Autodesk Inventor part; units mm, degrees
(part 2 of 2)
  arc A620 (20.4911, 0.6052) -> (20.4754, 1.0044) centre (0, 0) ccw
  arc A621 (20.3804, 2.2111) -> (20.3335, 2.6078) centre (0, 0) ccw
  arc A622 (20.1441, 3.8033) -> (20.0662, 4.1951) centre (0, 0) ccw
  arc A623 (19.7836, 5.372) -> (19.6752, 5.7565) centre (0, 0) ccw
  arc A624 (19.3011, 6.9077) -> (19.1629, 7.2825) centre (0, 0) ccw
  arc A625 (18.6997, 8.4007) -> (18.5324, 8.7635) centre (0, 0) ccw
  arc A626 (17.9829, 9.842) -> (17.7877, 10.1905) centre (0, 0) ccw
  arc A627 (17.1553, 11.2226) -> (16.9334, 11.5547) centre (0, 0) ccw
  arc A628 (16.2219, 12.534) -> (15.9746, 12.8477) centre (0, 0) ccw
  arc A629 (15.1885, 13.7681) -> (14.9173, 14.0614) centre (0, 0) ccw
  arc A630 (14.0614, 14.9173) -> (13.7681, 15.1885) centre (0, 0) ccw
  arc A631 (12.8477, 15.9746) -> (12.534, 16.2219) centre (0, 0) ccw
  arc A632 (11.5547, 16.9334) -> (11.2226, 17.1553) centre (0, 0) ccw
  arc A633 (10.1905, 17.7877) -> (9.842, 17.9829) centre (0, 0) ccw
  arc A634 (8.7635, 18.5324) -> (8.4007, 18.6997) centre (0, 0) ccw
  arc A635 (7.2825, 19.1629) -> (6.9077, 19.3011) centre (0, 0) ccw
  arc A636 (5.7565, 19.6752) -> (5.372, 19.7836) centre (0, 0) ccw
  arc A637 (4.1951, 20.0662) -> (3.8033, 20.1441) centre (0, 0) ccw
  arc A638 (2.6078, 20.3335) -> (2.2111, 20.3804) centre (0, 0) ccw
  arc A639 (1.0044, 20.4754) -> (0.6052, 20.4911) centre (0, 0) ccw
  line L0 (-22.5, 0) -> (22.5, 0)
  line L1 (0, -22.5) -> (0, 22.5)
  point P0 (0, 0)
  constraints: 960 point on circle, 480 centre point, 4 end point, 2 horizontal alignment, 2 vertical alignment, 1 horizontal, 1 vertical, 2081 other
extrude "押し出し1" add sketch "スケッチ1" along normal blind 3
sketch "スケッチ6" plane through (0, 0, 0) normal (0, 1, 0) x (-1, 0, 0)
  line L0 (0, 0) -> (0, 3)
  line L1 (0, 3) -> (-20, 3)
  line L2 (0, 0) -> (-20, 0)
  line L3 (-20, 3) -> (-20.5, 2.5)
  line L4 (-20.5, 2.5) -> (-20.5, 0.5)
  line L5 (-20.5, 0.5) -> (-20, 0)
  line L6 (-20, 3) -> (-20.5, 3)
  line L7 (-20.5, 3) -> (-20.5, 2.5)
  line L8 (-20, 0) -> (-20.5, 0)
  line L9 (-20.5, 0) -> (-20.5, 0.5)
  line L10 (0, 3) -> (0, 0)
  dimension "d30" = 3
  dimension "d31" = 0.5
  dimension "d32" = 0.5
  dimension "d33" = 0.5
  dimension "d34" = 0.5
  dimension "d35" = 20.5
  constraints: 22 end point, 4 horizontal, 3 vertical, 1 vertical alignment
  measures "d30" distance of L0.start L0.end
  measures "d31" horizontal distance of L1.end L3.end
  measures "d32" horizontal distance of L1.end L3.end
  measures "d33" horizontal distance of L4.end L2.end
  measures "d34" horizontal distance of L4.end L2.end
  measures "d35" distance from line of L0.start L4
revolve "回転1" cut sketch "スケッチ6" angle 360 about axis through (0, 0, 0) along (0, 0, 1) contours L8 L9 L5 | L3 L7 L6
sketch "スケッチ7" plane through (0, 0, 3) normal (0, 0, 1) x (1, 0, 0)
  circle A0 centre (0, 0) radius 17.25
  dimension "d37" = 34.5
  constraints: 1 centre point, 1 coincident
  measures "d37" diameter of A0
extrude "押し出し6" cut sketch "スケッチ7" against normal blind 0.8
sketch "スケッチ8" plane through (0, 0, 0) normal (0, 0, -1) x (-1, 0, 0)
  arc A0 (-0.3926, 19.9961) -> (-1.1774, 19.9653) centre (0, 0) ccw projected
  arc A1 (-1.1774, 19.9653) -> (-1.2665, 19.6357) centre (4.9618, 18.1301) ccw projected
  arc A2 (-1.2665, 19.6357) -> (-1.331, 19.3292) centre (3.8577, 18.3965) ccw projected
  arc A3 (-1.331, 19.3292) -> (-1.7091, 19.2995) centre (0, 0) ccw projected
  arc A4 (-1.7091, 19.2995) -> (-1.8197, 19.5895) centre (-6.6881, 17.5665) ccw projected
  arc A5 (-1.8197, 19.5895) -> (-1.9603, 19.9037) centre (-7.7369, 17.1307) ccw projected
  arc A6 (-1.9603, 19.9037) -> (-2.7403, 19.8114) centre (0, 0) ccw projected
  arc A7 (-2.7403, 19.8114) -> (-2.8032, 19.4758) centre (3.5241, 18.4635) ccw projected
  arc A8 (-2.8032, 19.4758) -> (-2.8435, 19.1652) centre (2.4025, 18.6425) ccw projected
  arc A9 (-2.8435, 19.1652) -> (-3.2181, 19.1059) centre (0, 0) ccw projected
  arc A10 (-3.2181, 19.1059) -> (-3.3511, 19.3863) centre (-8.0457, 16.9876) ccw projected
  arc A11 (-3.3511, 19.3863) -> (-3.5159, 19.6885) centre (-9.0571, 16.4708) ccw projected
  arc A12 (-3.5159, 19.6885) -> (-4.2862, 19.5353) centre (0, 0) ccw projected
  arc A13 (-4.2862, 19.5353) -> (-4.3226, 19.1958) centre (2.0646, 18.6831) ccw projected
  arc A14 (-4.3226, 19.1958) -> (-4.3384, 18.883) centre (0.9324, 18.7735) ccw projected
  arc A15 (-4.3384, 18.883) -> (-4.7072, 18.7945) centre (0, 0) ccw projected
  arc A16 (-4.7072, 18.7945) -> (-4.8632, 19.066) centre (-9.3537, 16.304) ccw projected
  arc A17 (-4.8632, 19.066) -> (-5.0498, 19.352) centre (-10.3215, 15.7095) ccw projected
  arc A18 (-5.0498, 19.352) -> (-5.8057, 19.1388) centre (0, 0) ccw projected
  arc A19 (-5.8057, 19.1388) -> (-5.8154, 18.7975) centre (0.5924, 18.7875) ccw projected
  arc A20 (-5.8154, 18.7975) -> (-5.8066, 18.4844) centre (-0.5434, 18.7888) ccw projected
  arc A21 (-5.8066, 18.4844) -> (-6.1673, 18.3672) centre (0, 0) ccw projected
  arc A22 (-6.1673, 18.3672) -> (-6.3442, 18.6257) centre (-10.6041, 15.5199) ccw projected
  arc A23 (-6.3442, 18.6257) -> (-6.5526, 18.8961) centre (-11.5222, 14.8512) ccw projected
  arc A24 (-6.5526, 18.8961) -> (-7.2894, 18.6243) centre (0, 0) ccw projected
  arc A25 (-7.2894, 18.6243) -> (-7.2723, 18.2833) centre (-0.8835, 18.776) ccw projected
  arc A26 (-7.2723, 18.2833) -> (-7.2389, 17.9719) centre (-2.0159, 18.6882) ccw projected
  arc A27 (-7.2389, 17.9719) -> (-7.5893, 17.8267) centre (0, 0) ccw projected
  arc A28 (-7.5893, 17.8267) -> (-7.786, 18.0705) centre (-11.7891, 14.64) ccw projected
  arc A29 (-7.786, 18.0705) -> (-8.0149, 18.3238) centre (-12.6519, 13.9014) ccw projected
  arc A30 (-8.0149, 18.3238) -> (-8.7282, 17.995) centre (0, 0) ccw projected
  arc A31 (-8.7282, 17.995) -> (-8.6843, 17.6563) centre (-2.3539, 18.6488) ccw projected
  arc A32 (-8.6843, 17.6563) -> (-8.6267, 17.3485) centre (-3.476, 18.4724) ccw projected
  arc A33 (-8.6267, 17.3485) -> (-8.9646, 17.1763) centre (0, 0) ccw projected
  arc A34 (-8.9646, 17.1763) -> (-9.1797, 17.4039) centre (-12.9014, 13.6699) ccw projected
  arc A35 (-9.1797, 17.4039) -> (-9.4279, 17.6384) centre (-13.7036, 12.8659) ccw projected
  arc A36 (-9.4279, 17.6384) -> (-10.1132, 17.2547) centre (0, 0) ccw projected
  arc A37 (-10.1132, 17.2547) -> (-10.0429, 16.9205) centre (-3.8099, 18.4067) ccw projected
  arc A38 (-10.0429, 16.9205) -> (-9.9612, 16.6182) centre (-4.9146, 18.1428) ccw projected
  arc A39 (-9.9612, 16.6182) -> (-10.2846, 16.42) centre (0, 0) ccw projected
  arc A40 (-10.2846, 16.42) -> (-10.5169, 16.63) centre (-13.9341, 12.6156) ccw projected
  arc A41 (-10.5169, 16.63) -> (-10.7827, 16.8444) centre (-14.6708, 11.7511) ccw projected
  arc A42 (-10.7827, 16.8444) -> (-11.4358, 16.408) centre (0, 0) ccw projected
  arc A43 (-11.4358, 16.408) -> (-11.3395, 16.0804) centre (-5.2423, 18.051) ccw projected
  arc A44 (-11.3395, 16.0804) -> (-11.2344, 15.7854) centre (-6.3229, 17.7012) ccw projected
  arc A45 (-11.2344, 15.7854) -> (-11.5412, 15.5625) centre (0, 0) ccw projected
  arc A46 (-11.5412, 15.5625) -> (-11.7893, 15.7536) centre (-14.881, 11.4834) ccw projected
  arc A47 (-11.7893, 15.7536) -> (-12.0711, 15.9464) centre (-15.5476, 10.5638) ccw projected
  arc A48 (-12.0711, 15.9464) -> (-12.6879, 15.4602) centre (0, 0) ccw projected
  arc A49 (-12.6879, 15.4602) -> (-12.5662, 15.1412) centre (-6.6424, 17.5841) ccw projected
  arc A50 (-12.5662, 15.1412) -> (-12.4383, 14.8553) centre (-7.6922, 17.1506) ccw projected
  arc A51 (-12.4383, 14.8553) -> (-12.7266, 14.609) centre (0, 0) ccw projected
  arc A52 (-12.7266, 14.609) -> (-12.989, 14.7801) centre (-15.7361, 10.2805) ccw projected
  arc A53 (-12.989, 14.7801) -> (-13.285, 14.9502) centre (-16.3285, 9.3114) ccw projected
  arc A54 (-13.285, 14.9502) -> (-13.8618, 14.417) centre (0, 0) ccw projected
  arc A55 (-13.8618, 14.417) -> (-13.7154, 14.1086) centre (-8.0015, 17.0087) ccw projected
  arc A56 (-13.7154, 14.1086) -> (-13.5655, 13.8336) centre (-9.0141, 16.4942) ccw projected
  arc A57 (-13.5655, 13.8336) -> (-13.8336, 13.5655) centre (0, 0) ccw projected
  arc A58 (-13.8336, 13.5655) -> (-14.1086, 13.7154) centre (-16.4942, 9.0141) ccw projected
  arc A59 (-14.1086, 13.7154) -> (-14.417, 13.8618) centre (-17.0087, 8.0015) ccw projected
  arc A60 (-14.417, 13.8618) -> (-14.9502, 13.285) centre (0, 0) ccw projected
  arc A61 (-14.9502, 13.285) -> (-14.7801, 12.989) centre (-9.3114, 16.3285) ccw projected
  arc A62 (-14.7801, 12.989) -> (-14.609, 12.7266) centre (-10.2805, 15.7361) ccw projected
  arc A63 (-14.609, 12.7266) -> (-14.8553, 12.4383) centre (0, 0) ccw projected
  arc A64 (-14.8553, 12.4383) -> (-15.1412, 12.5662) centre (-17.1506, 7.6922) ccw projected
  arc A65 (-15.1412, 12.5662) -> (-15.4602, 12.6879) centre (-17.5841, 6.6424) ccw projected
  arc A66 (-15.4602, 12.6879) -> (-15.9464, 12.0711) centre (0, 0) ccw projected
  arc A67 (-15.9464, 12.0711) -> (-15.7536, 11.7893) centre (-10.5638, 15.5476) ccw projected
  arc A68 (-15.7536, 11.7893) -> (-15.5625, 11.5412) centre (-11.4834, 14.881) ccw projected
  arc A69 (-15.5625, 11.5412) -> (-15.7854, 11.2344) centre (0, 0) ccw projected
  arc A70 (-15.7854, 11.2344) -> (-16.0804, 11.3395) centre (-17.7012, 6.3229) ccw projected
  arc A71 (-16.0804, 11.3395) -> (-16.408, 11.4358) centre (-18.051, 5.2423) ccw projected
  arc A72 (-16.408, 11.4358) -> (-16.8444, 10.7827) centre (0, 0) ccw projected
  arc A73 (-16.8444, 10.7827) -> (-16.63, 10.5169) centre (-11.7511, 14.6708) ccw projected
  arc A74 (-16.63, 10.5169) -> (-16.42, 10.2846) centre (-12.6156, 13.9341) ccw projected
  arc A75 (-16.42, 10.2846) -> (-16.6182, 9.9612) centre (0, 0) ccw projected
  arc A76 (-16.6182, 9.9612) -> (-16.9205, 10.0429) centre (-18.1428, 4.9146) ccw projected
  arc A77 (-16.9205, 10.0429) -> (-17.2547, 10.1132) centre (-18.4067, 3.8099) ccw projected
  arc A78 (-17.2547, 10.1132) -> (-17.6384, 9.4279) centre (0, 0) ccw projected
  arc A79 (-17.6384, 9.4279) -> (-17.4039, 9.1797) centre (-12.8659, 13.7036) ccw projected
  arc A80 (-17.4039, 9.1797) -> (-17.1763, 8.9646) centre (-13.6699, 12.9014) ccw projected
  arc A81 (-17.1763, 8.9646) -> (-17.3485, 8.6267) centre (0, 0) ccw projected
  arc A82 (-17.3485, 8.6267) -> (-17.6563, 8.6843) centre (-18.4724, 3.476) ccw projected
  arc A83 (-17.6563, 8.6843) -> (-17.995, 8.7282) centre (-18.6488, 2.3539) ccw projected
  arc A84 (-17.995, 8.7282) -> (-18.3238, 8.0149) centre (0, 0) ccw projected
  arc A85 (-18.3238, 8.0149) -> (-18.0705, 7.786) centre (-13.9014, 12.6519) ccw projected
  arc A86 (-18.0705, 7.786) -> (-17.8267, 7.5893) centre (-14.64, 11.7891) ccw projected
  arc A87 (-17.8267, 7.5893) -> (-17.9719, 7.2389) centre (0, 0) ccw projected
  arc A88 (-17.9719, 7.2389) -> (-18.2833, 7.2723) centre (-18.6882, 2.0159) ccw projected
  arc A89 (-18.2833, 7.2723) -> (-18.6243, 7.2894) centre (-18.776, 0.8835) ccw projected
  arc A90 (-18.6243, 7.2894) -> (-18.8961, 6.5526) centre (0, 0) ccw projected
  arc A91 (-18.8961, 6.5526) -> (-18.6234, 6.3425) centre (-14.8512, 11.5222) ccw projected
  arc A92 (-18.6234, 6.3425) -> (-18.3672, 6.1673) centre (-15.5198, 10.6041) ccw projected
  arc A93 (-18.3672, 6.1673) -> (-18.4844, 5.8066) centre (0, 0) ccw projected
  arc A94 (-18.4844, 5.8066) -> (-18.7975, 5.8154) centre (-18.7888, 0.5434) ccw projected
  arc A95 (-18.7975, 5.8154) -> (-19.1388, 5.8057) centre (-18.7875, -0.5924) ccw projected
  arc A96 (-19.1388, 5.8057) -> (-19.352, 5.0498) centre (0, 0) ccw projected
  arc A97 (-19.352, 5.0498) -> (-19.066, 4.8632) centre (-15.7095, 10.3215) ccw projected
  arc A98 (-19.066, 4.8632) -> (-18.7945, 4.7072) centre (-16.304, 9.3537) ccw projected
  arc A99 (-18.7945, 4.7072) -> (-18.883, 4.3384) centre (0, 0) ccw projected
  arc A100 (-18.883, 4.3384) -> (-19.1958, 4.3226) centre (-18.7735, -0.9324) ccw projected
  arc A101 (-19.1958, 4.3226) -> (-19.5353, 4.2862) centre (-18.6831, -2.0646) ccw projected
  arc A102 (-19.5353, 4.2862) -> (-19.6885, 3.5159) centre (0, 0) ccw projected
  arc A103 (-19.6885, 3.5159) -> (-19.3863, 3.3511) centre (-16.4708, 9.0571) ccw projected
  arc A104 (-19.3863, 3.3511) -> (-19.1059, 3.2181) centre (-16.9876, 8.0457) ccw projected
  arc A105 (-19.1059, 3.2181) -> (-19.1652, 2.8435) centre (0, 0) ccw projected
  arc A106 (-19.1652, 2.8435) -> (-19.4758, 2.8032) centre (-18.6425, -2.4025) ccw projected
  arc A107 (-19.4758, 2.8032) -> (-19.8114, 2.7403) centre (-18.4635, -3.5241) ccw projected
  arc A108 (-19.8114, 2.7403) -> (-19.9037, 1.9603) centre (0, 0) ccw projected
  arc A109 (-19.9037, 1.9603) -> (-19.592, 1.8208) centre (-17.1307, 7.7369) ccw projected
  arc A110 (-19.592, 1.8208) -> (-19.2995, 1.7091) centre (-17.5665, 6.6881) ccw projected
  arc A111 (-19.2995, 1.7091) -> (-19.3292, 1.331) centre (0, 0) ccw projected
  arc A112 (-19.3292, 1.331) -> (-19.6357, 1.2665) centre (-18.3965, -3.8577) ccw projected
  arc A113 (-19.6357, 1.2665) -> (-19.9653, 1.1774) centre (-18.1301, -4.9618) ccw projected
  arc A114 (-19.9653, 1.1774) -> (-19.9961, 0.3926) centre (0, 0) ccw projected
  arc A115 (-19.9961, 0.3926) -> (-19.6745, 0.278) centre (-17.6849, 6.369) ccw projected
  arc A116 (-19.6745, 0.278) -> (-19.3741, 0.1896) centre (-18.0371, 5.2892) ccw projected
  arc A117 (-19.3741, 0.1896) -> (-19.3741, -0.1896) centre (0, 0) ccw projected
  arc A118 (-19.3741, -0.1896) -> (-19.6745, -0.278) centre (-18.0371, -5.2892) ccw projected
  arc A119 (-19.6745, -0.278) -> (-19.9961, -0.3926) centre (-17.6849, -6.369) ccw projected
  arc A120 (-19.9961, -0.3926) -> (-19.9653, -1.1774) centre (0, 0) ccw projected
  arc A121 (-19.9653, -1.1774) -> (-19.6357, -1.2665) centre (-18.1301, 4.9618) ccw projected
  arc A122 (-19.6357, -1.2665) -> (-19.3292, -1.331) centre (-18.3965, 3.8577) ccw projected
  arc A123 (-19.3292, -1.331) -> (-19.2995, -1.7091) centre (0, 0) ccw projected
  arc A124 (-19.2995, -1.7091) -> (-19.592, -1.8208) centre (-17.5665, -6.6881) ccw projected
  arc A125 (-19.592, -1.8208) -> (-19.9037, -1.9603) centre (-17.1307, -7.7369) ccw projected
  arc A126 (-19.9037, -1.9603) -> (-19.8114, -2.7403) centre (0, 0) ccw projected
  arc A127 (-19.8114, -2.7403) -> (-19.4758, -2.8032) centre (-18.4635, 3.5241) ccw projected
  arc A128 (-19.4758, -2.8032) -> (-19.1652, -2.8435) centre (-18.6425, 2.4025) ccw projected
  arc A129 (-19.1652, -2.8435) -> (-19.1059, -3.2181) centre (0, 0) ccw projected
  arc A130 (-19.1059, -3.2181) -> (-19.3888, -3.3524) centre (-16.9876, -8.0457) ccw projected
  arc A131 (-19.3888, -3.3524) -> (-19.6885, -3.5159) centre (-16.4708, -9.0571) ccw projected
  arc A132 (-19.6885, -3.5159) -> (-19.5353, -4.2862) centre (0, 0) ccw projected
  arc A133 (-19.5353, -4.2862) -> (-19.1958, -4.3226) centre (-18.6831, 2.0646) ccw projected
  arc A134 (-19.1958, -4.3226) -> (-18.883, -4.3384) centre (-18.7735, 0.9324) ccw projected
  arc A135 (-18.883, -4.3384) -> (-18.7945, -4.7072) centre (0, 0) ccw projected
  arc A136 (-18.7945, -4.7072) -> (-19.066, -4.8632) centre (-16.304, -9.3537) ccw projected
  arc A137 (-19.066, -4.8632) -> (-19.352, -5.0498) centre (-15.7095, -10.3215) ccw projected
  arc A138 (-19.352, -5.0498) -> (-19.1388, -5.8057) centre (0, 0) ccw projected
  arc A139 (-19.1388, -5.8057) -> (-18.7975, -5.8154) centre (-18.7875, 0.5924) ccw projected
  arc A140 (-18.7975, -5.8154) -> (-18.4844, -5.8066) centre (-18.7888, -0.5434) ccw projected
  arc A141 (-18.4844, -5.8066) -> (-18.3672, -6.1673) centre (0, 0) ccw projected
  arc A142 (-18.3672, -6.1673) -> (-18.6257, -6.3442) centre (-15.5199, -10.6041) ccw projected
  arc A143 (-18.6257, -6.3442) -> (-18.8961, -6.5526) centre (-14.8512, -11.5222) ccw projected
  arc A144 (-18.8961, -6.5526) -> (-18.6243, -7.2894) centre (0, 0) ccw projected
  arc A145 (-18.6243, -7.2894) -> (-18.2833, -7.2723) centre (-18.776, -0.8835) ccw projected
  arc A146 (-18.2833, -7.2723) -> (-17.9719, -7.2389) centre (-18.6882, -2.0159) ccw projected
  arc A147 (-17.9719, -7.2389) -> (-17.8267, -7.5893) centre (0, 0) ccw projected
  arc A148 (-17.8267, -7.5893) -> (-18.0705, -7.786) centre (-14.64, -11.7891) ccw projected
  arc A149 (-18.0705, -7.786) -> (-18.3238, -8.0149) centre (-13.9014, -12.6519) ccw projected
  arc A150 (-18.3238, -8.0149) -> (-17.995, -8.7282) centre (0, 0) ccw projected
  arc A151 (-17.995, -8.7282) -> (-17.6563, -8.6843) centre (-18.6488, -2.3539) ccw projected
  arc A152 (-17.6563, -8.6843) -> (-17.3485, -8.6267) centre (-18.4724, -3.476) ccw projected
  arc A153 (-17.3485, -8.6267) -> (-17.1763, -8.9646) centre (0, 0) ccw projected
  arc A154 (-17.1763, -8.9646) -> (-17.4039, -9.1797) centre (-13.6699, -12.9014) ccw projected
  arc A155 (-17.4039, -9.1797) -> (-17.6384, -9.4279) centre (-12.8659, -13.7036) ccw projected
  arc A156 (-17.6384, -9.4279) -> (-17.2547, -10.1132) centre (0, 0) ccw projected
  arc A157 (-17.2547, -10.1132) -> (-16.9205, -10.0429) centre (-18.4067, -3.8099) ccw projected
  arc A158 (-16.9205, -10.0429) -> (-16.6182, -9.9612) centre (-18.1428, -4.9146) ccw projected
  arc A159 (-16.6182, -9.9612) -> (-16.42, -10.2846) centre (0, 0) ccw projected
  arc A160 (-16.42, -10.2846) -> (-16.6282, -10.5148) centre (-12.6156, -13.9341) ccw projected
  arc A161 (-16.6282, -10.5148) -> (-16.8444, -10.7827) centre (-11.7511, -14.6708) ccw projected
  arc A162 (-16.8444, -10.7827) -> (-16.408, -11.4358) centre (0, 0) ccw projected
  arc A163 (-16.408, -11.4358) -> (-16.0804, -11.3395) centre (-18.051, -5.2423) ccw projected
  arc A164 (-16.0804, -11.3395) -> (-15.7854, -11.2344) centre (-17.7012, -6.3229) ccw projected
  arc A165 (-15.7854, -11.2344) -> (-15.5625, -11.5412) centre (0, 0) ccw projected
  arc A166 (-15.5625, -11.5412) -> (-15.7536, -11.7893) centre (-11.4834, -14.881) ccw projected
  arc A167 (-15.7536, -11.7893) -> (-15.9464, -12.0711) centre (-10.5638, -15.5476) ccw projected
  arc A168 (-15.9464, -12.0711) -> (-15.4602, -12.6879) centre (0, 0) ccw projected
  arc A169 (-15.4602, -12.6879) -> (-15.1412, -12.5662) centre (-17.5841, -6.6424) ccw projected
  arc A170 (-15.1412, -12.5662) -> (-14.8553, -12.4383) centre (-17.1506, -7.6922) ccw projected
  arc A171 (-14.8553, -12.4383) -> (-14.609, -12.7266) centre (0, 0) ccw projected
  arc A172 (-14.609, -12.7266) -> (-14.7801, -12.989) centre (-10.2805, -15.7361) ccw projected
  arc A173 (-14.7801, -12.989) -> (-14.9502, -13.285) centre (-9.3114, -16.3285) ccw projected
  arc A174 (-14.9502, -13.285) -> (-14.417, -13.8618) centre (0, 0) ccw projected
  arc A175 (-14.417, -13.8618) -> (-14.1086, -13.7154) centre (-17.0087, -8.0015) ccw projected
  arc A176 (-14.1086, -13.7154) -> (-13.8336, -13.5655) centre (-16.4942, -9.0141) ccw projected
  arc A177 (-13.8336, -13.5655) -> (-13.5655, -13.8336) centre (0, 0) ccw projected
  arc A178 (-13.5655, -13.8336) -> (-13.7154, -14.1086) centre (-9.0141, -16.4942) ccw projected
  arc A179 (-13.7154, -14.1086) -> (-13.8618, -14.417) centre (-8.0015, -17.0087) ccw projected
  arc A180 (-13.8618, -14.417) -> (-13.285, -14.9502) centre (0, 0) ccw projected
  arc A181 (-13.285, -14.9502) -> (-12.989, -14.7801) centre (-16.3285, -9.3114) ccw projected
  arc A182 (-12.989, -14.7801) -> (-12.7266, -14.609) centre (-15.7361, -10.2805) ccw projected
  arc A183 (-12.7266, -14.609) -> (-12.4383, -14.8553) centre (0, 0) ccw projected
  arc A184 (-12.4383, -14.8553) -> (-12.5662, -15.1412) centre (-7.6922, -17.1506) ccw projected
  arc A185 (-12.5662, -15.1412) -> (-12.6879, -15.4602) centre (-6.6424, -17.5841) ccw projected
  arc A186 (-12.6879, -15.4602) -> (-12.0711, -15.9464) centre (0, 0) ccw projected
  arc A187 (-12.0711, -15.9464) -> (-11.7893, -15.7536) centre (-15.5476, -10.5638) ccw projected
  arc A188 (-11.7893, -15.7536) -> (-11.5412, -15.5625) centre (-14.881, -11.4834) ccw projected
  arc A189 (-11.5412, -15.5625) -> (-11.2344, -15.7854) centre (0, 0) ccw projected
  arc A190 (-11.2344, -15.7854) -> (-11.3386, -16.0778) centre (-6.3229, -17.7012) ccw projected
  arc A191 (-11.3386, -16.0778) -> (-11.4358, -16.408) centre (-5.2423, -18.051) ccw projected
  arc A192 (-11.4358, -16.408) -> (-10.7827, -16.8444) centre (0, 0) ccw projected
  arc A193 (-10.7827, -16.8444) -> (-10.5169, -16.63) centre (-14.6708, -11.7511) ccw projected
  arc A194 (-10.5169, -16.63) -> (-10.2846, -16.42) centre (-13.9341, -12.6156) ccw projected
  arc A195 (-10.2846, -16.42) -> (-9.9612, -16.6182) centre (0, 0) ccw projected
  arc A196 (-9.9612, -16.6182) -> (-10.0429, -16.9205) centre (-4.9146, -18.1428) ccw projected
  arc A197 (-10.0429, -16.9205) -> (-10.1132, -17.2547) centre (-3.8099, -18.4067) ccw projected
  arc A198 (-10.1132, -17.2547) -> (-9.4279, -17.6384) centre (0, 0) ccw projected
  arc A199 (-9.4279, -17.6384) -> (-9.1797, -17.4039) centre (-13.7036, -12.8659) ccw projected
  arc A200 (-9.1797, -17.4039) -> (-8.9646, -17.1763) centre (-12.9014, -13.6699) ccw projected
  arc A201 (-8.9646, -17.1763) -> (-8.6267, -17.3485) centre (0, 0) ccw projected
  arc A202 (-8.6267, -17.3485) -> (-8.6843, -17.6563) centre (-3.476, -18.4724) ccw projected
  arc A203 (-8.6843, -17.6563) -> (-8.7282, -17.995) centre (-2.3539, -18.6488) ccw projected
  arc A204 (-8.7282, -17.995) -> (-8.0149, -18.3238) centre (0, 0) ccw projected
  arc A205 (-8.0149, -18.3238) -> (-7.786, -18.0705) centre (-12.6519, -13.9014) ccw projected
  arc A206 (-7.786, -18.0705) -> (-7.5893, -17.8267) centre (-11.7891, -14.64) ccw projected
  arc A207 (-7.5893, -17.8267) -> (-7.2389, -17.9719) centre (0, 0) ccw projected
  arc A208 (-7.2389, -17.9719) -> (-7.2723, -18.2833) centre (-2.0159, -18.6882) ccw projected
  arc A209 (-7.2723, -18.2833) -> (-7.2894, -18.6243) centre (-0.8835, -18.776) ccw projected
  arc A210 (-7.2894, -18.6243) -> (-6.5526, -18.8961) centre (0, 0) ccw projected
  arc A211 (-6.5526, -18.8961) -> (-6.3442, -18.6257) centre (-11.5222, -14.8512) ccw projected
  arc A212 (-6.3442, -18.6257) -> (-6.1673, -18.3672) centre (-10.6041, -15.5199) ccw projected
  arc A213 (-6.1673, -18.3672) -> (-5.8066, -18.4844) centre (0, 0) ccw projected
  arc A214 (-5.8066, -18.4844) -> (-5.8154, -18.7975) centre (-0.5434, -18.7888) ccw projected
  arc A215 (-5.8154, -18.7975) -> (-5.8057, -19.1388) centre (0.5924, -18.7875) ccw projected
  arc A216 (-5.8057, -19.1388) -> (-5.0498, -19.352) centre (0, 0) ccw projected
  arc A217 (-5.0498, -19.352) -> (-4.8632, -19.066) centre (-10.3215, -15.7095) ccw projected
  arc A218 (-4.8632, -19.066) -> (-4.7072, -18.7945) centre (-9.3537, -16.304) ccw projected
  arc A219 (-4.7072, -18.7945) -> (-4.3384, -18.883) centre (0, 0) ccw projected
  arc A220 (-4.3384, -18.883) -> (-4.3226, -19.1958) centre (0.9324, -18.7735) ccw projected
  arc A221 (-4.3226, -19.1958) -> (-4.2862, -19.5353) centre (2.0646, -18.6831) ccw projected
  arc A222 (-4.2862, -19.5353) -> (-3.5159, -19.6885) centre (0, 0) ccw projected
  arc A223 (-3.5159, -19.6885) -> (-3.3524, -19.3888) centre (-9.0571, -16.4708) ccw projected
  arc A224 (-3.3524, -19.3888) -> (-3.2181, -19.1059) centre (-8.0457, -16.9876) ccw projected
  arc A225 (-3.2181, -19.1059) -> (-2.8435, -19.1652) centre (0, 0) ccw projected
  arc A226 (-2.8435, -19.1652) -> (-2.8032, -19.4758) centre (2.4025, -18.6425) ccw projected
  arc A227 (-2.8032, -19.4758) -> (-2.7403, -19.8114) centre (3.5241, -18.4635) ccw projected
  arc A228 (-2.7403, -19.8114) -> (-1.9603, -19.9037) centre (0, 0) ccw projected
  arc A229 (-1.9603, -19.9037) -> (-1.8208, -19.592) centre (-7.7369, -17.1307) ccw projected
  arc A230 (-1.8208, -19.592) -> (-1.7091, -19.2995) centre (-6.6881, -17.5665) ccw projected
  arc A231 (-1.7091, -19.2995) -> (-1.331, -19.3292) centre (0, 0) ccw projected
  arc A232 (-1.331, -19.3292) -> (-1.2665, -19.6357) centre (3.8577, -18.3965) ccw projected
  arc A233 (-1.2665, -19.6357) -> (-1.1774, -19.9653) centre (4.9618, -18.1301) ccw projected
  arc A234 (-1.1774, -19.9653) -> (-0.3926, -19.9961) centre (0, 0) ccw projected
  arc A235 (-0.3926, -19.9961) -> (-0.2771, -19.6719) centre (-6.369, -17.6849) ccw projected
  arc A236 (-0.2771, -19.6719) -> (-0.1896, -19.3741) centre (-5.2892, -18.0371) ccw projected
  arc A237 (-0.1896, -19.3741) -> (0.1896, -19.3741) centre (0, 0) ccw projected
  arc A238 (0.1896, -19.3741) -> (0.278, -19.6745) centre (5.2892, -18.0371) ccw projected
  arc A239 (0.278, -19.6745) -> (0.3926, -19.9961) centre (6.369, -17.6849) ccw projected
  arc A240 (0.3926, -19.9961) -> (1.1774, -19.9653) centre (0, 0) ccw projected
  arc A241 (1.1774, -19.9653) -> (1.2671, -19.633) centre (-4.9618, -18.1301) ccw projected
  arc A242 (1.2671, -19.633) -> (1.331, -19.3292) centre (-3.8577, -18.3965) ccw projected
  arc A243 (1.331, -19.3292) -> (1.7091, -19.2995) centre (0, 0) ccw projected
  arc A244 (1.7091, -19.2995) -> (1.8208, -19.592) centre (6.6881, -17.5665) ccw projected
  arc A245 (1.8208, -19.592) -> (1.9603, -19.9037) centre (7.7369, -17.1307) ccw projected
  arc A246 (1.9603, -19.9037) -> (2.7403, -19.8114) centre (0, 0) ccw projected
  arc A247 (2.7403, -19.8114) -> (2.8032, -19.4758) centre (-3.5241, -18.4635) ccw projected
  arc A248 (2.8032, -19.4758) -> (2.8435, -19.1652) centre (-2.4025, -18.6425) ccw projected
  arc A249 (2.8435, -19.1652) -> (3.2181, -19.1059) centre (0, 0) ccw projected
  arc A250 (3.2181, -19.1059) -> (3.3524, -19.3888) centre (8.0457, -16.9876) ccw projected
  arc A251 (3.3524, -19.3888) -> (3.5159, -19.6885) centre (9.0571, -16.4708) ccw projected
  arc A252 (3.5159, -19.6885) -> (4.2862, -19.5353) centre (0, 0) ccw projected
  arc A253 (4.2862, -19.5353) -> (4.3226, -19.1958) centre (-2.0646, -18.6831) ccw projected
  arc A254 (4.3226, -19.1958) -> (4.3384, -18.883) centre (-0.9324, -18.7735) ccw projected
  arc A255 (4.3384, -18.883) -> (4.7072, -18.7945) centre (0, 0) ccw projected
  arc A256 (4.7072, -18.7945) -> (4.8632, -19.066) centre (9.3537, -16.304) ccw projected
  arc A257 (4.8632, -19.066) -> (5.0498, -19.352) centre (10.3215, -15.7095) ccw projected
  arc A258 (5.0498, -19.352) -> (5.8057, -19.1388) centre (0, 0) ccw projected
  arc A259 (5.8057, -19.1388) -> (5.8154, -18.7975) centre (-0.5924, -18.7875) ccw projected
  arc A260 (5.8154, -18.7975) -> (5.8066, -18.4844) centre (0.5434, -18.7888) ccw projected
  arc A261 (5.8066, -18.4844) -> (6.1673, -18.3672) centre (0, 0) ccw projected
  arc A262 (6.1673, -18.3672) -> (6.3442, -18.6257) centre (10.6041, -15.5199) ccw projected
  arc A263 (6.3442, -18.6257) -> (6.5526, -18.8961) centre (11.5222, -14.8512) ccw projected
  arc A264 (6.5526, -18.8961) -> (7.2894, -18.6243) centre (0, 0) ccw projected
  arc A265 (7.2894, -18.6243) -> (7.272, -18.2805) centre (0.8835, -18.776) ccw projected
  arc A266 (7.272, -18.2805) -> (7.2389, -17.9719) centre (2.0159, -18.6882) ccw projected
  arc A267 (7.2389, -17.9719) -> (7.5893, -17.8267) centre (0, 0) ccw projected
  arc A268 (7.5893, -17.8267) -> (7.786, -18.0705) centre (11.7891, -14.64) ccw projected
  arc A269 (7.786, -18.0705) -> (8.0149, -18.3238) centre (12.6519, -13.9014) ccw projected
  arc A270 (8.0149, -18.3238) -> (8.7282, -17.995) centre (0, 0) ccw projected
  arc A271 (8.7282, -17.995) -> (8.6843, -17.6563) centre (2.3539, -18.6488) ccw projected
  arc A272 (8.6843, -17.6563) -> (8.6267, -17.3485) centre (3.476, -18.4724) ccw projected
  arc A273 (8.6267, -17.3485) -> (8.9646, -17.1763) centre (0, 0) ccw projected
  arc A274 (8.9646, -17.1763) -> (9.1797, -17.4039) centre (12.9014, -13.6699) ccw projected
  arc A275 (9.1797, -17.4039) -> (9.4279, -17.6384) centre (13.7036, -12.8659) ccw projected
  arc A276 (9.4279, -17.6384) -> (10.1132, -17.2547) centre (0, 0) ccw projected
  arc A277 (10.1132, -17.2547) -> (10.0429, -16.9205) centre (3.8099, -18.4067) ccw projected
  arc A278 (10.0429, -16.9205) -> (9.9612, -16.6182) centre (4.9146, -18.1428) ccw projected
  arc A279 (9.9612, -16.6182) -> (10.2846, -16.42) centre (0, 0) ccw projected
  arc A280 (10.2846, -16.42) -> (10.5169, -16.63) centre (13.9341, -12.6156) ccw projected
  arc A281 (10.5169, -16.63) -> (10.7827, -16.8444) centre (14.6708, -11.7511) ccw projected
  arc A282 (10.7827, -16.8444) -> (11.4358, -16.408) centre (0, 0) ccw projected
  arc A283 (11.4358, -16.408) -> (11.3395, -16.0804) centre (5.2423, -18.051) ccw projected
  arc A284 (11.3395, -16.0804) -> (11.2344, -15.7854) centre (6.3229, -17.7012) ccw projected
  arc A285 (11.2344, -15.7854) -> (11.5412, -15.5625) centre (0, 0) ccw projected
  arc A286 (11.5412, -15.5625) -> (11.7893, -15.7536) centre (14.881, -11.4834) ccw projected
  arc A287 (11.7893, -15.7536) -> (12.0711, -15.9464) centre (15.5476, -10.5638) ccw projected
  arc A288 (12.0711, -15.9464) -> (12.6879, -15.4602) centre (0, 0) ccw projected
  arc A289 (12.6879, -15.4602) -> (12.5662, -15.1412) centre (6.6424, -17.5841) ccw projected
  arc A290 (12.5662, -15.1412) -> (12.4383, -14.8553) centre (7.6922, -17.1506) ccw projected
  arc A291 (12.4383, -14.8553) -> (12.7266, -14.609) centre (0, 0) ccw projected
  arc A292 (12.7266, -14.609) -> (12.989, -14.7801) centre (15.7361, -10.2805) ccw projected
  arc A293 (12.989, -14.7801) -> (13.285, -14.9502) centre (16.3285, -9.3114) ccw projected
  arc A294 (13.285, -14.9502) -> (13.8618, -14.417) centre (0, 0) ccw projected
  arc A295 (13.8618, -14.417) -> (13.7154, -14.1086) centre (8.0015, -17.0087) ccw projected
  arc A296 (13.7154, -14.1086) -> (13.5655, -13.8336) centre (9.0141, -16.4942) ccw projected
  arc A297 (13.5655, -13.8336) -> (13.8336, -13.5655) centre (0, 0) ccw projected
  arc A298 (13.8336, -13.5655) -> (14.1086, -13.7154) centre (16.4942, -9.0141) ccw projected
  arc A299 (14.1086, -13.7154) -> (14.417, -13.8618) centre (17.0087, -8.0015) ccw projected
  arc A300 (14.417, -13.8618) -> (14.9502, -13.285) centre (0, 0) ccw projected
  arc A301 (14.9502, -13.285) -> (14.7801, -12.989) centre (9.3114, -16.3285) ccw projected
  arc A302 (14.7801, -12.989) -> (14.609, -12.7266) centre (10.2805, -15.7361) ccw projected
  arc A303 (14.609, -12.7266) -> (14.8553, -12.4383) centre (0, 0) ccw projected
  arc A304 (14.8553, -12.4383) -> (15.1412, -12.5662) centre (17.1506, -7.6922) ccw projected
  arc A305 (15.1412, -12.5662) -> (15.4602, -12.6879) centre (17.5841, -6.6424) ccw projected
  arc A306 (15.4602, -12.6879) -> (15.9464, -12.0711) centre (0, 0) ccw projected
  arc A307 (15.9464, -12.0711) -> (15.7536, -11.7893) centre (10.5638, -15.5476) ccw projected
  arc A308 (15.7536, -11.7893) -> (15.5625, -11.5412) centre (11.4834, -14.881) ccw projected
  arc A309 (15.5625, -11.5412) -> (15.7854, -11.2344) centre (0, 0) ccw projected
  arc A310 (15.7854, -11.2344) -> (16.0778, -11.3386) centre (17.7012, -6.3229) ccw projected
  arc A311 (16.0778, -11.3386) -> (16.408, -11.4358) centre (18.051, -5.2423) ccw projected
  arc A312 (16.408, -11.4358) -> (16.8444, -10.7827) centre (0, 0) ccw projected
  arc A313 (16.8444, -10.7827) -> (16.63, -10.5169) centre (11.7511, -14.6708) ccw projected
  arc A314 (16.63, -10.5169) -> (16.42, -10.2846) centre (12.6156, -13.9341) ccw projected
  arc A315 (16.42, -10.2846) -> (16.6182, -9.9612) centre (0, 0) ccw projected
  arc A316 (16.6182, -9.9612) -> (16.9205, -10.0429) centre (18.1428, -4.9146) ccw projected
  arc A317 (16.9205, -10.0429) -> (17.2547, -10.1132) centre (18.4067, -3.8099) ccw projected
  arc A318 (17.2547, -10.1132) -> (17.6384, -9.4279) centre (0, 0) ccw projected
  arc A319 (17.6384, -9.4279) -> (17.4039, -9.1797) centre (12.8659, -13.7036) ccw projected
  arc A320 (17.4039, -9.1797) -> (17.1763, -8.9646) centre (13.6699, -12.9014) ccw projected
  arc A321 (17.1763, -8.9646) -> (17.3485, -8.6267) centre (0, 0) ccw projected
  arc A322 (17.3485, -8.6267) -> (17.6563, -8.6843) centre (18.4724, -3.476) ccw projected
  arc A323 (17.6563, -8.6843) -> (17.995, -8.7282) centre (18.6488, -2.3539) ccw projected
  arc A324 (17.995, -8.7282) -> (18.3238, -8.0149) centre (0, 0) ccw projected
  arc A325 (18.3238, -8.0149) -> (18.0705, -7.786) centre (13.9014, -12.6519) ccw projected
  arc A326 (18.0705, -7.786) -> (17.8267, -7.5893) centre (14.64, -11.7891) ccw projected
  arc A327 (17.8267, -7.5893) -> (17.9719, -7.2389) centre (0, 0) ccw projected
  arc A328 (17.9719, -7.2389) -> (18.2833, -7.2723) centre (18.6882, -2.0159) ccw projected
  arc A329 (18.2833, -7.2723) -> (18.6243, -7.2894) centre (18.776, -0.8835) ccw projected
  arc A330 (18.6243, -7.2894) -> (18.8961, -6.5526) centre (0, 0) ccw projected
  arc A331 (18.8961, -6.5526) -> (18.6234, -6.3425) centre (14.8512, -11.5222) ccw projected
  arc A332 (18.6234, -6.3425) -> (18.3672, -6.1673) centre (15.5199, -10.6041) ccw projected
  arc A333 (18.3672, -6.1673) -> (18.4844, -5.8066) centre (0, 0) ccw projected
  arc A334 (18.4844, -5.8066) -> (18.7975, -5.8154) centre (18.7888, -0.5434) ccw projected
  arc A335 (18.7975, -5.8154) -> (19.1388, -5.8057) centre (18.7875, 0.5924) ccw projected
  arc A336 (19.1388, -5.8057) -> (19.352, -5.0498) centre (0, 0) ccw projected
  arc A337 (19.352, -5.0498) -> (19.066, -4.8632) centre (15.7095, -10.3215) ccw projected
  arc A338 (19.066, -4.8632) -> (18.7945, -4.7072) centre (16.304, -9.3537) ccw projected
  arc A339 (18.7945, -4.7072) -> (18.883, -4.3384) centre (0, 0) ccw projected
  arc A340 (18.883, -4.3384) -> (19.1958, -4.3226) centre (18.7735, 0.9324) ccw projected
  arc A341 (19.1958, -4.3226) -> (19.5353, -4.2862) centre (18.6831, 2.0646) ccw projected
  arc A342 (19.5353, -4.2862) -> (19.6885, -3.5159) centre (0, 0) ccw projected
  arc A343 (19.6885, -3.5159) -> (19.3888, -3.3524) centre (16.4708, -9.0571) ccw projected
  arc A344 (19.3888, -3.3524) -> (19.1059, -3.2181) centre (16.9876, -8.0457) ccw projected
  arc A345 (19.1059, -3.2181) -> (19.1652, -2.8435) centre (0, 0) ccw projected
  arc A346 (19.1652, -2.8435) -> (19.4758, -2.8032) centre (18.6425, 2.4025) ccw projected
  arc A347 (19.4758, -2.8032) -> (19.8114, -2.7403) centre (18.4635, 3.5241) ccw projected
  arc A348 (19.8114, -2.7403) -> (19.9037, -1.9603) centre (0, 0) ccw projected
  arc A349 (19.9037, -1.9603) -> (19.592, -1.8208) centre (17.1307, -7.7369) ccw projected
  arc A350 (19.592, -1.8208) -> (19.2995, -1.7091) centre (17.5665, -6.6881) ccw projected
  arc A351 (19.2995, -1.7091) -> (19.3292, -1.331) centre (0, 0) ccw projected
  arc A352 (19.3292, -1.331) -> (19.6357, -1.2665) centre (18.3965, 3.8577) ccw projected
  arc A353 (19.6357, -1.2665) -> (19.9653, -1.1774) centre (18.1301, 4.9618) ccw projected
  arc A354 (19.9653, -1.1774) -> (19.9961, -0.3926) centre (0, 0) ccw projected
  arc A355 (19.9961, -0.3926) -> (19.6745, -0.278) centre (17.6849, -6.369) ccw projected
  arc A356 (19.6745, -0.278) -> (19.3741, -0.1896) centre (18.0371, -5.2892) ccw projected
  arc A357 (19.3741, -0.1896) -> (19.3741, 0.1896) centre (0, 0) ccw projected
  arc A358 (19.3741, 0.1896) -> (19.6745, 0.278) centre (18.0371, 5.2892) ccw projected
  arc A359 (19.6745, 0.278) -> (19.9961, 0.3926) centre (17.6849, 6.369) ccw projected
  arc A360 (19.9961, 0.3926) -> (19.9653, 1.1774) centre (0, 0) ccw projected
  arc A361 (19.9653, 1.1774) -> (19.6357, 1.2665) centre (18.1301, -4.9618) ccw projected
  arc A362 (19.6357, 1.2665) -> (19.3292, 1.331) centre (18.3965, -3.8577) ccw projected
  arc A363 (19.3292, 1.331) -> (19.2995, 1.7091) centre (0, 0) ccw projected
  arc A364 (19.2995, 1.7091) -> (19.592, 1.8208) centre (17.5665, 6.6881) ccw projected
  arc A365 (19.592, 1.8208) -> (19.9037, 1.9603) centre (17.1307, 7.7369) ccw projected
  arc A366 (19.9037, 1.9603) -> (19.8114, 2.7403) centre (0, 0) ccw projected
  arc A367 (19.8114, 2.7403) -> (19.4758, 2.8032) centre (18.4635, -3.5241) ccw projected
  arc A368 (19.4758, 2.8032) -> (19.1652, 2.8435) centre (18.6425, -2.4025) ccw projected
  arc A369 (19.1652, 2.8435) -> (19.1059, 3.2181) centre (0, 0) ccw projected
  arc A370 (19.1059, 3.2181) -> (19.3888, 3.3524) centre (16.9876, 8.0457) ccw projected
  arc A371 (19.3888, 3.3524) -> (19.6885, 3.5159) centre (16.4708, 9.0571) ccw projected
  arc A372 (19.6885, 3.5159) -> (19.5353, 4.2862) centre (0, 0) ccw projected
  arc A373 (19.5353, 4.2862) -> (19.1958, 4.3226) centre (18.6831, -2.0646) ccw projected
  arc A374 (19.1958, 4.3226) -> (18.883, 4.3384) centre (18.7735, -0.9324) ccw projected
  arc A375 (18.883, 4.3384) -> (18.7945, 4.7072) centre (0, 0) ccw projected
  arc A376 (18.7945, 4.7072) -> (19.066, 4.8632) centre (16.304, 9.3537) ccw projected
  arc A377 (19.066, 4.8632) -> (19.352, 5.0498) centre (15.7095, 10.3215) ccw projected
  arc A378 (19.352, 5.0498) -> (19.1388, 5.8057) centre (0, 0) ccw projected
  arc A379 (19.1388, 5.8057) -> (18.7975, 5.8154) centre (18.7875, -0.5924) ccw projected
  arc A380 (18.7975, 5.8154) -> (18.4844, 5.8066) centre (18.7888, 0.5434) ccw projected
  arc A381 (18.4844, 5.8066) -> (18.3672, 6.1673) centre (0, 0) ccw projected
  arc A382 (18.3672, 6.1673) -> (18.6257, 6.3442) centre (15.5199, 10.6041) ccw projected
  arc A383 (18.6257, 6.3442) -> (18.8961, 6.5526) centre (14.8512, 11.5222) ccw projected
  arc A384 (18.8961, 6.5526) -> (18.6243, 7.2894) centre (0, 0) ccw projected
  arc A385 (18.6243, 7.2894) -> (18.2805, 7.272) centre (18.776, 0.8835) ccw projected
  arc A386 (18.2805, 7.272) -> (17.9719, 7.2389) centre (18.6882, 2.0159) ccw projected
  arc A387 (17.9719, 7.2389) -> (17.8267, 7.5893) centre (0, 0) ccw projected
  arc A388 (17.8267, 7.5893) -> (18.0705, 7.786) centre (14.64, 11.7891) ccw projected
  arc A389 (18.0705, 7.786) -> (18.3238, 8.0149) centre (13.9014, 12.6519) ccw projected
  arc A390 (18.3238, 8.0149) -> (17.995, 8.7282) centre (0, 0) ccw projected
  arc A391 (17.995, 8.7282) -> (17.6536, 8.6839) centre (18.6488, 2.3539) ccw projected
  arc A392 (17.6536, 8.6839) -> (17.3485, 8.6267) centre (18.4724, 3.476) ccw projected
  arc A393 (17.3485, 8.6267) -> (17.1763, 8.9646) centre (0, 0) ccw projected
  arc A394 (17.1763, 8.9646) -> (17.4039, 9.1797) centre (13.6699, 12.9014) ccw projected
  arc A395 (17.4039, 9.1797) -> (17.6384, 9.4279) centre (12.8659, 13.7036) ccw projected
  arc A396 (17.6384, 9.4279) -> (17.2547, 10.1132) centre (0, 0) ccw projected
  arc A397 (17.2547, 10.1132) -> (16.9205, 10.0429) centre (18.4067, 3.8099) ccw projected
  arc A398 (16.9205, 10.0429) -> (16.6182, 9.9612) centre (18.1428, 4.9146) ccw projected
  arc A399 (16.6182, 9.9612) -> (16.42, 10.2846) centre (0, 0) ccw projected
  arc A400 (16.42, 10.2846) -> (16.63, 10.5169) centre (12.6156, 13.9341) ccw projected
  arc A401 (16.63, 10.5169) -> (16.8444, 10.7827) centre (11.7511, 14.6708) ccw projected
  arc A402 (16.8444, 10.7827) -> (16.408, 11.4358) centre (0, 0) ccw projected
  arc A403 (16.408, 11.4358) -> (16.0804, 11.3395) centre (18.051, 5.2423) ccw projected
  arc A404 (16.0804, 11.3395) -> (15.7854, 11.2344) centre (17.7012, 6.3229) ccw projected
  arc A405 (15.7854, 11.2344) -> (15.5625, 11.5412) centre (0, 0) ccw projected
  arc A406 (15.5625, 11.5412) -> (15.7536, 11.7893) centre (11.4834, 14.881) ccw projected
  arc A407 (15.7536, 11.7893) -> (15.9464, 12.0711) centre (10.5638, 15.5476) ccw projected
  arc A408 (15.9464, 12.0711) -> (15.4602, 12.6879) centre (0, 0) ccw projected
  arc A409 (15.4602, 12.6879) -> (15.1412, 12.5662) centre (17.5841, 6.6424) ccw projected
  arc A410 (15.1412, 12.5662) -> (14.8553, 12.4383) centre (17.1506, 7.6922) ccw projected
  arc A411 (14.8553, 12.4383) -> (14.609, 12.7266) centre (0, 0) ccw projected
  arc A412 (14.609, 12.7266) -> (14.7801, 12.989) centre (10.2805, 15.7361) ccw projected
  arc A413 (14.7801, 12.989) -> (14.9502, 13.285) centre (9.3114, 16.3285) ccw projected
  arc A414 (14.9502, 13.285) -> (14.417, 13.8618) centre (0, 0) ccw projected
  arc A415 (14.417, 13.8618) -> (14.1086, 13.7154) centre (17.0087, 8.0015) ccw projected
  arc A416 (14.1086, 13.7154) -> (13.8336, 13.5655) centre (16.4942, 9.0141) ccw projected
  arc A417 (13.8336, 13.5655) -> (13.5655, 13.8336) centre (0, 0) ccw projected
  arc A418 (13.5655, 13.8336) -> (13.7154, 14.1086) centre (9.0141, 16.4942) ccw projected
  arc A419 (13.7154, 14.1086) -> (13.8618, 14.417) centre (8.0015, 17.0087) ccw projected
  arc A420 (13.8618, 14.417) -> (13.285, 14.9502) centre (0, 0) ccw projected
  arc A421 (13.285, 14.9502) -> (12.989, 14.7801) centre (16.3285, 9.3114) ccw projected
  arc A422 (12.989, 14.7801) -> (12.7266, 14.609) centre (15.7361, 10.2805) ccw projected
  arc A423 (12.7266, 14.609) -> (12.4383, 14.8553) centre (0, 0) ccw projected
  arc A424 (12.4383, 14.8553) -> (12.5662, 15.1412) centre (7.6922, 17.1506) ccw projected
  arc A425 (12.5662, 15.1412) -> (12.6879, 15.4602) centre (6.6424, 17.5841) ccw projected
  arc A426 (12.6879, 15.4602) -> (12.0711, 15.9464) centre (0, 0) ccw projected
  arc A427 (12.0711, 15.9464) -> (11.7893, 15.7536) centre (15.5476, 10.5638) ccw projected
  arc A428 (11.7893, 15.7536) -> (11.5412, 15.5625) centre (14.881, 11.4834) ccw projected
  arc A429 (11.5412, 15.5625) -> (11.2344, 15.7854) centre (0, 0) ccw projected
  arc A430 (11.2344, 15.7854) -> (11.3395, 16.0804) centre (6.3229, 17.7012) ccw projected
  arc A431 (11.3395, 16.0804) -> (11.4358, 16.408) centre (5.2423, 18.051) ccw projected
  arc A432 (11.4358, 16.408) -> (10.7827, 16.8444) centre (0, 0) ccw projected
  arc A433 (10.7827, 16.8444) -> (10.5169, 16.63) centre (14.6708, 11.7511) ccw projected
  arc A434 (10.5169, 16.63) -> (10.2846, 16.42) centre (13.9341, 12.6156) ccw projected
  arc A435 (10.2846, 16.42) -> (9.9612, 16.6182) centre (0, 0) ccw projected
  arc A436 (9.9612, 16.6182) -> (10.0429, 16.9205) centre (4.9146, 18.1428) ccw projected
  arc A437 (10.0429, 16.9205) -> (10.1132, 17.2547) centre (3.8099, 18.4067) ccw projected
  arc A438 (10.1132, 17.2547) -> (9.4279, 17.6384) centre (0, 0) ccw projected
  arc A439 (9.4279, 17.6384) -> (9.1778, 17.4019) centre (13.7036, 12.8659) ccw projected
  arc A440 (9.1778, 17.4019) -> (8.9646, 17.1763) centre (12.9014, 13.6699) ccw projected
  arc A441 (8.9646, 17.1763) -> (8.6267, 17.3485) centre (0, 0) ccw projected
  arc A442 (8.6267, 17.3485) -> (8.6843, 17.6563) centre (3.476, 18.4724) ccw projected
  arc A443 (8.6843, 17.6563) -> (8.7282, 17.995) centre (2.3539, 18.6488) ccw projected
  arc A444 (8.7282, 17.995) -> (8.0149, 18.3238) centre (0, 0) ccw projected
  arc A445 (8.0149, 18.3238) -> (7.786, 18.0705) centre (12.6519, 13.9014) ccw projected
  arc A446 (7.786, 18.0705) -> (7.5893, 17.8267) centre (11.7891, 14.64) ccw projected
  arc A447 (7.5893, 17.8267) -> (7.2389, 17.9719) centre (0, 0) ccw projected
  arc A448 (7.2389, 17.9719) -> (7.2723, 18.2833) centre (2.0159, 18.6882) ccw projected
  arc A449 (7.2723, 18.2833) -> (7.2894, 18.6243) centre (0.8835, 18.776) ccw projected
  arc A450 (7.2894, 18.6243) -> (6.5526, 18.8961) centre (0, 0) ccw projected
  arc A451 (6.5526, 18.8961) -> (6.3442, 18.6257) centre (11.5222, 14.8512) ccw projected
  arc A452 (6.3442, 18.6257) -> (6.1673, 18.3672) centre (10.6041, 15.5199) ccw projected
  arc A453 (6.1673, 18.3672) -> (5.8066, 18.4844) centre (0, 0) ccw projected
  arc A454 (5.8066, 18.4844) -> (5.8154, 18.7975) centre (0.5434, 18.7888) ccw projected
  arc A455 (5.8154, 18.7975) -> (5.8057, 19.1388) centre (-0.5924, 18.7875) ccw projected
  arc A456 (5.8057, 19.1388) -> (5.0498, 19.352) centre (0, 0) ccw projected
  arc A457 (5.0498, 19.352) -> (4.8632, 19.066) centre (10.3215, 15.7095) ccw projected
  arc A458 (4.8632, 19.066) -> (4.7072, 18.7945) centre (9.3537, 16.304) ccw projected
  arc A459 (4.7072, 18.7945) -> (4.3384, 18.883) centre (0, 0) ccw projected
  arc A460 (4.3384, 18.883) -> (4.3226, 19.1958) centre (-0.9324, 18.7735) ccw projected
  arc A461 (4.3226, 19.1958) -> (4.2862, 19.5353) centre (-2.0646, 18.6831) ccw projected
  arc A462 (4.2862, 19.5353) -> (3.5159, 19.6885) centre (0, 0) ccw projected
  arc A463 (3.5159, 19.6885) -> (3.3524, 19.3888) centre (9.0571, 16.4708) ccw projected
  arc A464 (3.3524, 19.3888) -> (3.2181, 19.1059) centre (8.0457, 16.9876) ccw projected
  arc A465 (3.2181, 19.1059) -> (2.8435, 19.1652) centre (0, 0) ccw projected
  arc A466 (2.8435, 19.1652) -> (2.8032, 19.4758) centre (-2.4025, 18.6425) ccw projected
  arc A467 (2.8032, 19.4758) -> (2.7403, 19.8114) centre (-3.5241, 18.4635) ccw projected
  arc A468 (2.7403, 19.8114) -> (1.9603, 19.9037) centre (0, 0) ccw projected
  arc A469 (1.9603, 19.9037) -> (1.8197, 19.5895) centre (7.7369, 17.1307) ccw projected
  arc A470 (1.8197, 19.5895) -> (1.7091, 19.2995) centre (6.6881, 17.5665) ccw projected
  arc A471 (1.7091, 19.2995) -> (1.331, 19.3292) centre (0, 0) ccw projected
  arc A472 (1.331, 19.3292) -> (1.2665, 19.6357) centre (-3.8577, 18.3965) ccw projected
  arc A473 (1.2665, 19.6357) -> (1.1774, 19.9653) centre (-4.9618, 18.1301) ccw projected
  arc A474 (1.1774, 19.9653) -> (0.3926, 19.9961) centre (0, 0) ccw projected
  arc A475 (0.3926, 19.9961) -> (0.2771, 19.6719) centre (6.369, 17.6849) ccw projected
  arc A476 (0.2771, 19.6719) -> (0.1896, 19.3741) centre (5.2892, 18.0371) ccw projected
  arc A477 (0.1896, 19.3741) -> (-0.1896, 19.3741) centre (0, 0) ccw projected
  arc A478 (-0.1896, 19.3741) -> (-0.278, 19.6745) centre (-5.2892, 18.0371) ccw projected
  arc A479 (-0.278, 19.6745) -> (-0.3926, 19.9961) centre (-6.369, 17.6849) ccw projected
  circle A480 centre (0, 0) radius 17.3
  dimension "d40" = 34.6
  constraints: 1 centre point, 1 coincident
  measures "d40" diameter of A480
extrude "押し出し7" cut sketch "スケッチ8" against normal blind 0.5 contours A480
sketch "スケッチ9" plane through (0, 0, 2.2) normal (0, 0, 1) x (1, 0, 0)
  line L0 (0, 12) -> (10.3923, -6)
  line L1 (10.3923, -6) -> (-10.3923, -6)
  line L2 (-10.3923, -6) -> (0, 12)
  circle A0 centre (-10.3923, -6) radius 1.5
  circle A1 centre (10.3923, -6) radius 1.5
  circle A2 centre (0, 12) radius 1.5
  circle A3 centre (-10.3923, -6) radius 4.5
  circle A4 centre (0, 12) radius 4.5
  circle A5 centre (10.3923, -6) radius 4.5
  circle A6 centre (0, 0) radius 16.5
  circle A7 centre (0, 12) radius 4.5
  circle A8 centre (0, 0) radius 12
  point P0 (-4.4202, 11.1562)
  point P1 (-11.8717, -1.7501)
  point P2 (-7.4515, -9.4061)
  point P3 (7.4515, -9.4061)
  point P4 (11.8717, -1.7501)
  point P5 (4.4202, 11.1563)
  dimension "d43" = 3
  dimension "d44" = 3
  dimension "d45" = 3
  dimension "d46" = 9
  dimension "d47" = 9
  dimension "d48" = 9
  dimension "d49" = 33
  dimension "d50" = 9
  dimension "d51" = 24
  constraints: 10 coincident, 9 centre point, 6 end point, 1 horizontal, 1 tangent, 7 other
  measures "d43" diameter of A0
  measures "d44" diameter of A1
  measures "d45" diameter of A2
  measures "d46" diameter of A3
  measures "d47" diameter of A4
  measures "d48" diameter of A5
  measures "d49" diameter of A6
  measures "d50" diameter of A7
  measures "d51" diameter of A8
extrude "押し出し8" cut sketch "スケッチ9" against normal through all contours A8 A2 L0 | L0 A2 L2 | A8 A2 | L2 A2 A8 | A4 A8 A5 L0 | L0 A5 L1 A3 L2 A4 | L2 A3 A8 A4 | A1 A8 L0 | L0 L1 A1 | A5 A8 A3 L1 | A0 L1 L2 | L2 A8 A0 | A8 A0 | A8 A1 L1 | A8 A1 | L1 A0 A8
fillet "フィレット2" radius 2 6 edges at (-7.4515, -9.4061, 1.35) (-11.8717, -1.7501, 1.35) (-4.4202, 11.1562, 1.35) (4.4202, 11.1563, 1.35) (11.8717, -1.7501, 1.35) (7.4515, -9.4061, 1.35)
equation "\"d32\" = d31"
equation "\"d33\" = d31"
equation "\"d34\" = d31"
